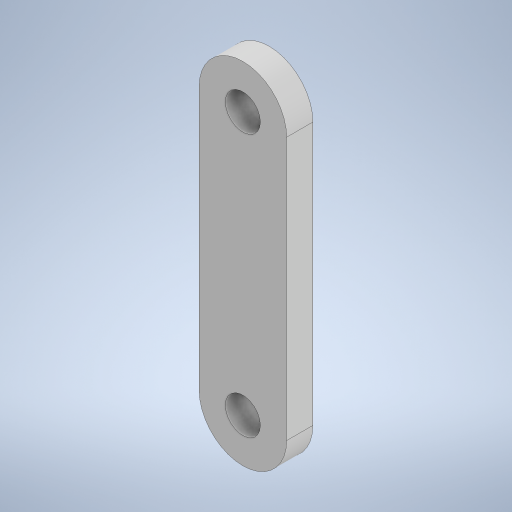
# Autodesk Inventor part: 13_Riostra
Saved by Autodesk Inventor 2024.3 (Build 283343000, 343)
## iProperties
Created: 2024-04-24
Part Number: 13_Riostra
Material: Genérico
Document SubType Name: Modeling
Designer: Cosmic Dinodog
Density: 1 g/cm^3
Appearance: Valor por defecto
Author: Cosmic Dinodog
Autodesk Inventor part; units mm, degrees
ref_plane "YZ Plane" through (0, 0, 0) normal (1, 0, 0) x (0, 1, 0)
ref_plane "XZ Plane" through (0, 0, 0) normal (0, 1, 0) x (-1, 0, 0)
ref_plane "XY Plane" through (0, 0, 0) normal (0, 0, 1) x (1, 0, 0)
sketch "Boceto1" plane through (0, 0, 0) normal (0, 0, 1) x (1, 0, 0)
  circle A0 centre (0, 0) radius 4
  arc A1 (-10, 0) -> (10, 0) centre (0, 0) ccw
  line L0 (0, 0) -> (0, 60) construction
  circle A2 centre (0, 60) radius 4
  arc A3 (10, 60) -> (-10, 60) centre (0, 60) ccw
  line L1 (-10, 60) -> (-10, 0)
  line L2 (10, 60) -> (10, 0)
  dimension "d0" = 8
  dimension "d1" = 20
  dimension "d2" = 60
  dimension "d3" = 8
  dimension "d4" = 20
  constraints: 6 end point, 4 centre point, 4 coincident, 4 point on circle, 4 tangent, 1 vertical
  measures "d0" diameter of A0
  measures "d1" diameter of A1
  measures "d2" distance of L0.start L0.end
  measures "d3" diameter of A2
  measures "d4" diameter of A3
extrude "Extrusión1" add sketch "Boceto1" against normal blind 6
